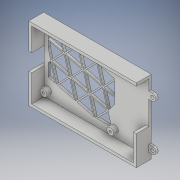
# Autodesk Inventor part: Deck
Saved by Autodesk Inventor 2019 (Build 230136000, 136)
## iProperties
Created: 2020-04-10
Part Number: Deck
Material: Generic
Document SubType Name: Modeling
Designer: Jorge
Density: 1 g/cm^3
Appearance: Default
Author: Jorge
Autodesk Inventor part; units mm, degrees
ref_plane "YZ Plane" through (0, 0, 0) normal (1, 0, 0) x (0, 1, 0)
ref_plane "XZ Plane" through (0, 0, 0) normal (0, 1, 0) x (-1, 0, 0)
ref_plane "XY Plane" through (0, 0, 0) normal (0, 0, 1) x (1, 0, 0)
sketch "Sketch1" plane through (0, 0, 0) normal (0, 0, 1) x (1, 0, 0)
  circle A0 centre (5.7, 58) radius 1
  circle A1 centre (63.7, 58) radius 1
  circle A2 centre (5.7, 9) radius 1
  circle A3 centre (63.7, 9) radius 1
  line L0 (5.7, 58) -> (63.7, 58) construction
  line L1 (63.7, 58) -> (63.7, 9) construction
  line L2 (63.7, 9) -> (5.7, 9) construction
  line L3 (5.7, 9) -> (5.7, 58) construction
  circle A4 centre (5.7, 58) radius 3
  circle A5 centre (63.7, 58) radius 3
  circle A6 centre (63.7, 9) radius 3
  circle A7 centre (5.7, 9) radius 3
  line L4 (2.5, 61.2) -> (93.2, 61.2)
  line L5 (93.2, 61.2) -> (93.2, 0)
  line L6 (2.5, 61.2) -> (93.2, 61.2)
  line L7 (93.2, 61.2) -> (93.2, 63.7)
  line L8 (93.2, 63.7) -> (2.5, 63.7)
  line L9 (2.5, 63.7) -> (2.5, 61.2)
  line L10 (2.5, 63.7) -> (0, 63.7)
  line L11 (0, 63.7) -> (0, 0)
  line L12 (2.5, 2.5) -> (2.5, 63.7)
  line L13 (0, 41) -> (2.5, 41)
  line L14 (2.5, 41) -> (2.5, 26)
  line L15 (2.5, 26) -> (0, 26)
  line L16 (0, 26) -> (0, 41)
  line L17 (5.7, 33.5) -> (0, 33.5) construction
  line L18 (2.5, 2.5) -> (90.7, 2.5)
  line L19 (93.2, -3.283) -> (93.2, 0)
  line L20 (93.2, 0) -> (0, 0)
  line L21 (2.5, 2.5) -> (2.5, 61.2)
  line L22 (93.2, 0) -> (62.7076, 0)
  line L23 (90.7, 2.5) -> (90.7, 25.5)
  line L24 (90.7, 25.5) -> (93.2, 25.5)
  line L25 (93.2, 25.5) -> (93.2, 0)
  line L26 (0, 49) -> (-3, 49) construction
  circle A8 centre (-3, 49) radius 1.5
  arc A9 (-3, 52) -> (-3, 46) centre (-3, 49) ccw
  line L27 (-3, 52) -> (-3, 46) construction
  line L28 (-3, 52) -> (0, 52)
  line L29 (-3, 46) -> (0, 46)
  line L30 (93.2, 49) -> (96.2, 49) construction
  circle A10 centre (96.2, 49) radius 1.5
  arc A11 (96.2, 46) -> (96.2, 52) centre (96.2, 49) ccw
  line L31 (96.2, 52) -> (96.2, 46) construction
  line L32 (96.2, 52) -> (93.2, 52)
  line L33 (96.2, 46) -> (93.2, 46)
  line L34 (0, 9) -> (-3, 9) construction
  circle A12 centre (-3, 9) radius 1.5
  arc A13 (-3, 12) -> (-3, 6) centre (-3, 9) ccw
  line L35 (-3, 12) -> (-3, 6) construction
  line L36 (-3, 12) -> (0, 12)
  line L37 (-3, 6) -> (0, 6)
  line L38 (93.2, 9) -> (96.2, 9) construction
  circle A14 centre (96.2, 9) radius 1.5
  arc A15 (96.2, 6) -> (96.2, 12) centre (96.2, 9) ccw
  line L39 (96.2, 6) -> (96.2, 12) construction
  line L40 (96.2, 12) -> (93.2, 12)
  line L41 (96.2, 6) -> (93.2, 6)
  line L42 (0, 41) -> (2.5, 41)
  line L43 (2.5, 41) -> (2.5, 63.7)
  line L44 (2.5, 63.7) -> (0, 63.7)
  line L45 (0, 63.7) -> (0, 41)
  line L46 (93.2, 0) -> (0, 0)
  line L47 (0, 0) -> (0, 2.5)
  line L48 (0, 2.5) -> (93.2, 2.5)
  line L49 (93.2, 2.5) -> (93.2, 0)
  line L50 (0, 0) -> (2.5, 0)
  line L51 (2.5, 0) -> (2.5, 26)
  line L52 (2.5, 26) -> (0, 26)
  line L53 (0, 26) -> (0, 0)
  line L54 (93.2, 25.5) -> (90.7, 25.5)
  line L55 (90.7, 25.5) -> (90.7, 0)
  line L56 (90.7, 0) -> (93.2, 0)
  line L57 (93.2, 0) -> (93.2, 25.5)
  line L58 (0, 41) -> (2.5, 41)
  line L59 (2.5, 41) -> (2.5, 63.7)
  line L60 (2.5, 63.7) -> (0, 63.7)
  line L61 (0, 63.7) -> (0, 41)
  line L62 (2.5, 41) -> (0, 41)
  line L63 (0, 41) -> (0, 26)
  line L64 (0, 26) -> (2.5, 26)
  line L65 (2.5, 26) -> (2.5, 41)
  dimension "d0" = 2
  dimension "d1" = 2
  dimension "d2" = 58
  dimension "d3" = 2
  dimension "d4" = 2
  dimension "d5" = 49
  dimension "d6" = 6
  dimension "d7" = 6
  dimension "d8" = 6
  dimension "d9" = 6
  dimension "d10" = 3.2
  dimension "d11" = 2.5
  dimension "d14" = 15
  dimension "d17" = 6.5
  dimension "d18" = 2.5
  dimension "d19" = 29.5
  dimension "d20" = 3.2
  dimension "d21" = 2.5
  dimension "d22" = 16.5
  dimension "d23" = 3
  dimension "d24" = 3
  dimension "d25" = 6
  dimension "d26" = 3
  dimension "d27" = 3
  dimension "d28" = 6
  dimension "d29" = 9
  dimension "d30" = 3
  dimension "d31" = 6
  dimension "d32" = 3
  dimension "d33" = 3
  dimension "d34" = 6
  dimension "d35" = 2.5
  dimension "d36" = 3
  dimension "d41" = 2.5
  dimension "d42" = 2.5
  constraints: 130 end point, 22 parallel, 20 perpendicular, 19 horizontal, 16 centre point, 14 coincident, 10 point on line, 8 point on circle, 7 midpoint, 4 vertical, 3 collinear, 1 symmetric about line, 12 other
  measures "d0" diameter of A0
  measures "d1" diameter of A1
  measures "d2" distance of A1.centre L0.start
  measures "d3" diameter of A2
  measures "d4" diameter of A3
  measures "d5" distance of A2.centre L0.start
  measures "d6" diameter of A4
  measures "d7" diameter of A5
  measures "d8" diameter of A6
  measures "d9" diameter of A7
  measures "d10" distance between parallel lines of L4 L0
  measures "d11" distance of L7.end L6.end
  measures "d14" distance of L13.end L14.end
  measures "d17" distance between parallel lines of L2 L18
  measures "d18" distance of the line from the sketch origin of L21
  measures "d19" distance between parallel lines of L5 L1
  measures "d20" distance between parallel lines of L21 L3
  measures "d21" distance of L23.end L24.end
  measures "d22" distance between parallel lines of L24 L2
  measures "d23" distance of L26.start L26.end
  measures "d24" diameter of A8
  measures "d25" distance between parallel lines of L28 L29
  measures "d26" distance of L30.start L30.end
  measures "d27" diameter of A10
  measures "d28" distance between parallel lines of L32 L33
  measures "d29" distance between parallel lines of L0 L26
  measures "d30" diameter of A12
  measures "d31" distance between parallel lines of L37 L36
  measures "d32" distance of L38.start L38.end
  measures "d33" diameter of A14
  measures "d34" distance between parallel lines of L40 L41
  measures "d35" distance between parallel lines of L20 L18
  measures "d36" distance of L34.start L34.end
  measures "d41" distance between parallel lines of L5 L55
  measures "d42" distance between parallel lines of L20 L48
extrude "Extrusion1" add sketch "Sketch1" along normal blind 2 contours A4 | A5 | A6 | A7 | L9 L8 L7 L4 | L12 L13 L11 L10 L9 | L4 L5 L24 L23 L18 L12 | L12 L15 L11 L13 | L32 A11 L33 L5 | L12 L48 L11 L15 | L11 L29 A9 L28 | L51 L20 L11 L48 | L18 L55 L20 L51 | L5 L48 L23 L24 | L48 L5 L20 L55 | L11 L37 A13 L36 | L40 A15 L41 L5
extrude "Extrusion2" add sketch "Sketch1" along normal blind 6 contours A4 | A5 | A6 | A7
extrude "Extrusion3" add sketch "Sketch1" along normal blind 13 contours L9 L8 L7 L4 | L12 L13 L11 L10 L9 | L12 L15 L11 L13 | L12 L48 L11 L15 | L51 L20 L11 L48 | L18 L55 L20 L51 | L5 L48 L23 L24 | L48 L5 L20 L55
extrude "Extrusion4" cut sketch "Sketch1" along normal blind 13 contours L12 L15 L11 L13
sketch "Sketch2" plane through (0, 0, 0) normal (0, 0, 1) x (1, 0, 0)
  line L0 (5.7, 47.7749) -> (51.6652, 36.1467) construction
  line L1 (5.7, 47.7749) -> (18.7571, 44.4717)
  line L2 (5.7, 51.2424) -> (12.2708, 58)
  line L3 (14.1282, 58) -> (18.7571, 44.4717)
  line L4 (20.8899, 43.9322) -> (35.4318, 40.2534)
  line L5 (35.4318, 40.2534) -> (31.3467, 54.6864)
  line L6 (31.3467, 54.6864) -> (20.8899, 43.9322)
  line L7 (37.5646, 39.7139) -> (52.1065, 36.0351)
  line L8 (52.1065, 36.0351) -> (48.0214, 50.4681)
  line L9 (48.0214, 50.4681) -> (37.5646, 39.7139)
  line L10 (54.2393, 35.4955) -> (63.7, 33.1022)
  line L11 (63.7, 45.2253) -> (54.2393, 35.4955)
  line L12 (18.2484, 58) -> (63.7, 46.5018) construction
  line L13 (18.2484, 58) -> (30.2803, 54.9562)
  line L14 (30.2803, 54.9562) -> (19.8235, 44.2019)
  line L15 (15.1183, 58) -> (19.8235, 44.2019)
  line L16 (32.4131, 54.4167) -> (46.955, 50.7379)
  line L17 (46.955, 50.7379) -> (36.4982, 39.9836)
  line L18 (32.4131, 54.4167) -> (36.4982, 39.9836)
  line L19 (49.0878, 50.1983) -> (63.6297, 46.5196)
  line L20 (63.6297, 46.5196) -> (53.1729, 35.7653)
  line L21 (53.1729, 35.7653) -> (49.0878, 50.1983)
  line L22 (5.7, 47.2833) -> (63.7, 32.6107) construction
  line L23 (5.7, 46.7918) -> (51.4315, 35.2228) construction
  line L24 (5.7, 46.7918) -> (18.5233, 43.5478)
  line L25 (5.7, 41.1547) -> (8.0665, 32.7936)
  line L26 (8.0665, 32.7936) -> (18.5233, 43.5478)
  line L27 (20.6562, 43.0083) -> (35.1981, 39.3295)
  line L28 (35.1981, 39.3295) -> (24.7412, 28.5752)
  line L29 (24.7412, 28.5752) -> (20.6562, 43.0083)
  line L30 (37.3309, 38.79) -> (51.8728, 35.1112)
  line L31 (51.8728, 35.1112) -> (41.4159, 24.3569)
  line L32 (41.4159, 24.3569) -> (37.3309, 38.79)
  line L33 (54.0056, 34.5716) -> (63.7, 32.1192)
  line L34 (63.7, 27.4724) -> (58.0906, 20.1386)
  line L35 (58.0906, 20.1386) -> (54.0056, 34.5716)
  line L36 (8.0665, 32.7936) -> (58.0906, 20.1386) construction
  line L37 (9.1329, 32.5238) -> (23.6748, 28.845)
  line L38 (23.6748, 28.845) -> (19.5898, 43.278)
  line L39 (9.1329, 32.5238) -> (19.5898, 43.278)
  line L40 (25.8076, 28.3055) -> (40.3495, 24.6267)
  line L41 (40.3495, 24.6267) -> (36.2645, 39.0597)
  line L42 (25.8076, 28.3055) -> (36.2645, 39.0597)
  line L43 (42.4823, 24.0872) -> (57.0242, 20.4084)
  line L44 (57.0242, 20.4084) -> (52.9392, 34.8414)
  line L45 (52.9392, 34.8414) -> (42.4823, 24.0872)
  line L46 (63.7, 18.2281) -> (5.7, 32.9007) construction
  line L47 (24.5075, 27.6513) -> (14.0506, 16.8971)
  line L48 (23.4411, 27.9211) -> (12.9842, 17.1669)
  line L49 (8.8992, 31.5999) -> (23.4411, 27.9211)
  line L50 (7.8328, 31.8697) -> (11.9178, 17.4366)
  line L51 (28.5925, 13.2183) -> (24.5075, 27.6513)
  line L52 (14.0506, 16.8971) -> (28.5925, 13.2183)
  line L53 (25.5739, 27.3816) -> (29.6589, 12.9485)
  line L54 (7.8328, 31.8697) -> (57.8569, 19.2147) construction
  line L55 (25.5739, 27.3816) -> (40.1158, 23.7028)
  line L56 (40.1158, 23.7028) -> (29.6589, 12.9485)
  line L57 (8.8992, 31.5999) -> (12.9842, 17.1669)
  line L58 (5.7, 29.6762) -> (7.8328, 31.8697)
  line L59 (5.7, 19.0096) -> (11.9178, 17.4366)
  line L60 (30.7253, 12.6788) -> (45.2672, 9)
  line L61 (46.2573, 9) -> (42.2486, 23.1633)
  line L62 (42.2486, 23.1633) -> (56.7905, 19.4845)
  line L63 (56.7905, 19.4845) -> (46.596, 9)
  line L64 (57.8569, 19.2147) -> (47.9247, 9)
  line L65 (60.748, 9) -> (57.8569, 19.2147)
  line L66 (41.1822, 23.433) -> (30.7253, 12.6788)
  line L67 (5.7, 58) -> (63.7, 58) construction
  line L68 (5.7, 9) -> (5.7, 58) construction
  line L69 (63.7, 9) -> (5.7, 9) construction
  line L70 (63.7, 58) -> (63.7, 9) construction
  line L71 (5.7, 29.6762) -> (5.7, 19.0096)
  line L72 (46.2573, 9) -> (46.596, 9)
  line L73 (60.748, 9) -> (47.9247, 9)
  line L74 (63.7, 32.1192) -> (63.7, 27.4724)
  line L75 (63.7, 45.2253) -> (63.7, 33.1022)
  line L76 (15.1183, 58) -> (18.2484, 58)
  line L77 (12.2708, 58) -> (14.1282, 58)
  line L78 (5.7, 41.1547) -> (5.7, 46.7918)
  line L79 (5.7, 51.2424) -> (5.7, 47.7749)
  line L80 (45.2672, 9) -> (41.1822, 23.433)
  point P0 (0, 0)
  point P1 (45.2672, 9)
  dimension "d62" = 15
  dimension "d63" = 15
  dimension "d64" = 15
  dimension "i_v" = 2.2
  dimension "d66" = 15
  dimension "d67" = 15
  dimension "d68" = 15
  dimension "d69" = 2.2
  dimension "d73" = 2.2
  dimension "d75" = 15
  dimension "d76" = 1.1
  dimension "d77" = 15
  dimension "d78" = 1.1
  dimension "d79" = 15
  dimension "d81" = 15
  dimension "d82" = 15
  dimension "d83" = 15
  dimension "d84" = 1.1
  dimension "d85" = 0.953
  dimension "d86" = 60
  dimension "d87" = 0.953
  dimension "d88" = 15
  dimension "d90" = 60
  dimension "d91" = 60
  dimension "d92" = 60
  dimension "d93" = 1.1
  dimension "d94" = 60
  dimension "d95" = 60
  dimension "d96" = 1.1
  dimension "d97" = 60
  constraints: 150 end point, 34 symmetric about line, 22 point on line, 4 collinear, 4 parallel, 3 vertical, 2 perpendicular, 51 other
  measures "d62" distance of L4.start L4.end
  measures "d63" distance of L4.end L5.end
  measures "d64" distance of L4.start L5.end
  measures "i_v" distance of L4.start L1.end
  measures "d66" distance of L7.start L7.end
  measures "d67" distance of L7.end L8.end
  measures "d68" distance of L7.start L8.end
  measures "d69" distance of L7.start L4.end
  measures "d73" distance of L7.end L10.start
  measures "d75" distance of L16.start L16.end
  measures "d76" distance of L4.start L14.end
  measures "d77" distance of L13.end L14.end
  measures "d78" distance of L17.end L4.end
  measures "d79" distance of L16.end L17.end
  measures "d81" distance of L19.start L19.end
  measures "d82" distance of L19.start L20.end
  measures "d83" distance of L19.end L20.end
  measures "d84" distance of L10.start L20.end
  measures "d85" distance between parallel lines of L10 L33
  measures "d86" angle of L10 L11
  measures "d88" distance of L66.end L60.end
  measures "d90" angle of L62 L61
  measures "d92" angle of L65 L64
  measures "d93" distance of L36.end L43.end
  measures "d94" angle of L50 L58
  measures "d95" angle of L26 L25
  measures "d96" distance of L49.start L50.start
  measures "d97" angle of L50 L59
extrude "Extrusion5" cut sketch "Sketch2" along normal blind 13
body "Solid1"
